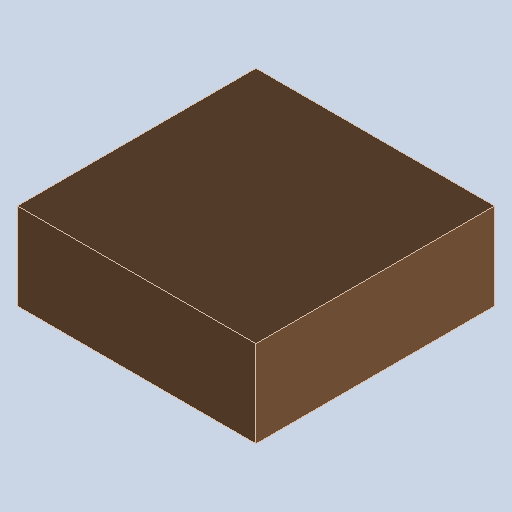
# Autodesk Inventor part: body
Saved by Autodesk Inventor 2025 (Build 290162000, 162)
## iProperties
Created: 2025-09-09
Part Number: body
Material: capacitor ceramic
Document SubType Name: Modeling
Designer: jirne
Density: 1 g/cm^3
Appearance: Generic
Author: jirne
Autodesk Inventor part; units mm, degrees
ref_plane "YZ Plane" through (0, 0, 0) normal (1, 0, 0) x (0, 1, 0)
ref_plane "XZ Plane" through (0, 0, 0) normal (0, 1, 0) x (-1, 0, 0)
ref_plane "XY Plane" through (0, 0, 0) normal (0, 0, 1) x (1, 0, 0)
sketch "Sketch1" plane through (0, 0, 0) normal (0, 0, 1) x (1, 0, 0)
  line L0 (0, 0) -> (2.794, 0)
  line L1 (2.794, 0) -> (2.794, 2.794)
  line L2 (2.794, 2.794) -> (0, 2.794)
  line L3 (0, 2.794) -> (0, 0)
  dimension "d0" = 2.794
  dimension "d1" = 2.794
  constraints: 8 end point, 2 parallel, 1 horizontal, 1 perpendicular
  measures "d0" distance of L0.end L1.end
  measures "d1" distance of L1.end L2.end
extrude "Extrusion1" add sketch "Sketch1" along normal blind 1.016
body "Solid1"
